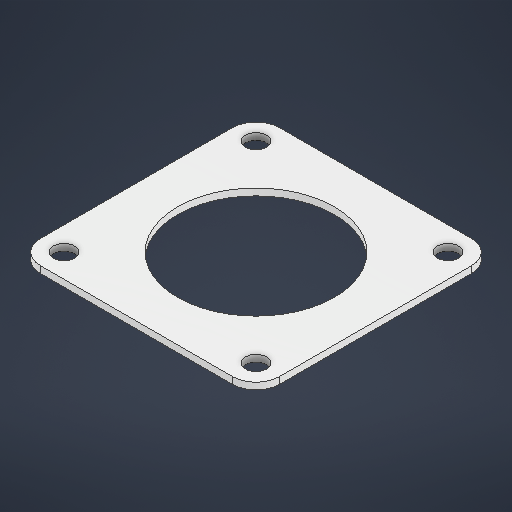
# Autodesk Inventor part: CNC-004-Nema23Shim
Saved by Autodesk Inventor 2026.2 (Build 302298000, 298)
## iProperties
Created: 2026-06-15
Part Number: CNC-004-Nema23Shim
Material: ABS Plastic
Document SubType Name: Modeling
Designer: Kenji
Density: 1.06 g/cm^3
Appearance: Smooth - White
Author: Kenji
Autodesk Inventor part; units mm, degrees
ref_plane "YZ Plane" through (0, 0, 0) normal (1, 0, 0) x (0, 1, 0)
ref_plane "XZ Plane" through (0, 0, 0) normal (0, 1, 0) x (-1, 0, 0)
ref_plane "XY Plane" through (0, 0, 0) normal (0, 0, 1) x (1, 0, 0)
sketch "Sketch1" plane through (0, 0, 0) normal (0, 1, 0) x (-1, 0, 0)
  circle A0 centre (0, 0) radius 19.25
  circle A1 centre (23.57, -23.57) radius 2.6
  circle A2 centre (23.57, 23.57) radius 2.6
  circle A3 centre (-23.57, 23.57) radius 2.6
  circle A4 centre (-23.57, -23.57) radius 2.6
  circle A5 centre (23.57, 23.57) radius 5.775 construction
  circle A6 centre (23.57, -23.57) radius 5.775 construction
  circle A7 centre (-23.57, -23.57) radius 5.775 construction
  circle A8 centre (-23.57, 23.57) radius 5.775 construction
  line L0 (29.345, 23.57) -> (29.345, -23.57)
  line L1 (23.57, -29.345) -> (-23.57, -29.345)
  line L2 (-29.345, -23.57) -> (-29.345, 23.57)
  line L3 (-23.57, 29.345) -> (23.57, 29.345)
  arc A9 (-29.345, -23.57) -> (-23.57, -29.345) centre (-23.57, -23.57) ccw
  arc A10 (-23.57, 29.345) -> (-29.345, 23.57) centre (-23.57, 23.57) ccw
  arc A11 (23.57, -29.345) -> (29.345, -23.57) centre (23.57, -23.57) ccw
  arc A12 (29.345, 23.57) -> (23.57, 29.345) centre (23.57, 23.57) ccw
  dimension "d0" = 38.5
  dimension "d1" = 5.2
  dimension "d2" = 23.57
  dimension "d3" = 23.57
  dimension "d4" = 23.57
  dimension "d5" = 23.57
  dimension "d6" = 3.175
  constraints: 17 point on circle, 13 centre point, 9 tangent, 8 end point, 8 equal radius, 4 coincident, 2 horizontal alignment, 2 vertical alignment, 1 perpendicular, 1 vertical
  measures "d0" diameter of A0
  measures "d1" diameter of A1
  measures "d2" horizontal distance of point (0, 0) A1.centre
  measures "d3" horizontal distance of point (0, 0) A1.centre
  measures "d4" horizontal distance of point (0, 0) A3.centre
  measures "d5" horizontal distance of point (0, 0) A3.centre
  measures "d6" radial gap between concentric circles of A5 A2
extrude "Extrusion1" add sketch "Sketch1" along normal blind 1.6625
body "Solid1"
